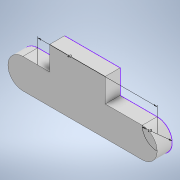
# Autodesk Inventor part: Part1
Saved by Autodesk Inventor 2022 (Build 260153000, 153)
## iProperties
Created: 2022-03-14
Part Number: Part1
Material: Generic
Document SubType Name: Modeling
Designer: br4ch
Density: 1 g/cm^3
Appearance: Default
Author: br4ch
Autodesk Inventor part; units mm, degrees
ref_plane "YZ Plane" through (0, 0, 0) normal (1, 0, 0) x (0, 1, 0)
ref_plane "XZ Plane" through (0, 0, 0) normal (0, 1, 0) x (-1, 0, 0)
ref_plane "XY Plane" through (0, 0, 0) normal (0, 0, 1) x (1, 0, 0)
sketch "Sketch1" plane through (0, 0, 0) normal (0, 0, 1) x (1, 0, 0)
  line L0 (-20, 3) -> (20, 3) construction
  line L1 (-20, -2) -> (20, -2)
  line L2 (20, 8) -> (-20, 8)
  arc A0 (-20, 8) -> (-20, -2) centre (-20, 3) ccw
  arc A1 (20, -2) -> (20, 8) centre (20, 3) ccw
  line L3 (-11, 16) -> (7.6141, 16)
  line L4 (7.6141, 16) -> (7.6141, 8)
  line L5 (7.6141, 8) -> (-11, 8)
  line L6 (-11, 8) -> (-11, 16)
  point P0 (0, 0)
  point P1 (0, 3)
  dimension "d0" = 10
  dimension "d2" = 40
  constraints: 16 end point, 4 point on circle, 4 tangent, 3 parallel, 2 centre point, 2 horizontal, 1 midpoint, 1 perpendicular, 1 point on line
  measures "d0" diameter of A1
  measures "d2" distance of L0.end L0.start
extrude "Extrusion1" add sketch "Sketch1" along normal blind 5 contours A0 L2 A1 L1
extrude "Extrusion3" add sketch "Sketch1" along normal blind 5 contours L6 L3 L4 L2
body "Solid1"
